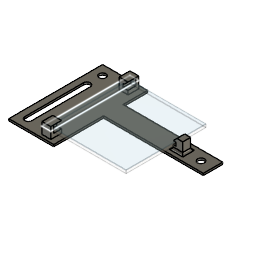
MDB-Slave-PCB-Holder (Autodesk Fusion 360 design; units mm, degrees)
Autodesk Fusion 360 part; units mm, degrees
sketch "Skizze1" plane through (0, 0, 0) normal (0, 0, 1) x (1, 0, 0) in component "Component"
  line L0 (19.5, -20.5) -> (-19.5, -20.5)
  line L1 (-19.5, -20.5) -> (-19.5, 20.5)
  line L2 (-19.5, 20.5) -> (19.5, 20.5)
  line L3 (19.5, 20.5) -> (19.5, -20.5)
  line L4 (19.5, -20.5) -> (-19.5, 20.5) construction
  line L5 (-19.5, -20.5) -> (19.5, 20.5) construction
  dimension "d19" = 39
  dimension "d20" = 41
  constraint horizontal L0
  constraint perpendicular L0 L1
  constraint parallel L0 L2
  constraint parallel L1 L3
  constraint coincident L4 origin
  constraint coincident L5 origin
  measures "d19" distance of L1.end L2.end
  measures "d20" distance of L0.end L1.end
extrude "Extrusion1" add sketch "Skizze1" along normal blind 1.7 makes body 1 in component "Component"
sketch "Skizze1 (2)" plane through (0, 0, 1.7) normal (0, 0, 1) x (-1, 0, 0) in component "Component'"
  line L0 (-19.5, -20.5) -> (19.5, -20.5)
  line L1 (19.5, -20.5) -> (19.5, 20.5)
  line L2 (19.5, 20.5) -> (-19.5, 20.5)
  line L3 (-19.5, 20.5) -> (-19.5, -20.5)
  line L4 (17, -22.5) -> (21.5, -22.5)
  line L5 (21.5, -22.5) -> (21.5, 22.5)
  line L6 (21.5, 22.5) -> (17, 22.5)
  line L7 (17, 22.5) -> (17, -22.5)
  dimension "d23" = 2
  dimension "d24" = 2
  dimension "d25" = 2.5
  dimension "d26" = 2
  constraint horizontal L4
  constraint vertical L5
  constraint horizontal L6
  constraint vertical L7
  measures "d23" distance of L2 L6
  measures "d24" distance of L0 L4
  measures "d25" distance of L1 L7
  measures "d26" distance of L1 L5
extrude "Extrusion1'" add sketch "Skizze1 (2)" against normal up to surface (1.7 mm away) separate body contours L0 L1 L2 L4 L5 L6 L7 makes body 2 in component "Component'"
extrude "Extrusion2" add sketch "Skizze1 (2)" along normal blind 1 separate body contours L0 L1 L2 L7 | L0 L1 L2 L4 L5 L6 L7 makes body 3 in component "Component'"
sketch "Skizze2" plane through (0, 0, 0) normal (0, 0, -1) x (1, 0, 0) in component "Component'"
  line L0 (-21.5, -22.5) -> (-17, -22.5)
  line L1 (-17, -22.5) -> (-17, -20.5)
  line L2 (-17, -20.5) -> (-19.5, -20.5)
  line L3 (-19.5, -20.5) -> (-19.5, 20.5)
  line L4 (-19.5, 20.5) -> (-17, 20.5)
  line L5 (-17, 20.5) -> (-17, 22.5)
  line L6 (-17, 22.5) -> (-21.5, 22.5)
  line L7 (-21.5, 22.5) -> (-21.5, -22.5)
  line L8 (-17, -20.5) -> (-17, 20.5)
  constraint coincident L1.end L2.start
  constraint coincident L4.end L5.start
extrude "Extrusion3" add sketch "Skizze2" along normal blind 2 bodies 2 in component "Component'"
sketch "Skizze3" plane through (0, 0, -2) normal (0, 0, -1) x (1, 0, 0) in component "Component'"
  line L0 (-17, -22.5) -> (-17, 22.5)
  line L1 (-17, 22.5) -> (-21.5, 22.5)
  line L2 (-21.5, 22.5) -> (-21.5, -22.5)
  line L3 (-21.5, -22.5) -> (-17, -22.5)
  line L4 (27, -24) -> (-27, -24)
  line L5 (-27, -24) -> (-27, 24)
  line L6 (-27, 24) -> (27, 24)
  line L7 (27, 24) -> (27, -24)
  line L8 (27, -24) -> (-27, 24) construction
  line L9 (-27, -24) -> (27, 24) construction
  constraint horizontal L4
  constraint perpendicular L4 L5
  constraint parallel L4 L6
  constraint parallel L5 L7
  constraint coincident L8 origin
  constraint coincident L9 origin
extrude "Extrusion4" add sketch "Skizze3" along normal blind 1 contours L0 L1 L2 L3 | L4 L5 L6 L7 bodies 2 in component "Component'"
sketch "Skizze4" plane through (0, 0, -2) normal (0, 0, 1) x (-1, 0, 0) in component "Component'"
  line L0 (27, 24) -> (-27, 24)
  line L1 (-27, 24) -> (-27, -24)
  line L2 (-27, -24) -> (27, -24)
  line L3 (27, -24) -> (27, 24)
  line L4 (21.5, -22.5) -> (17, -22.5)
  line L5 (17, -22.5) -> (17, 22.5)
  line L6 (17, 22.5) -> (21.5, 22.5)
  line L7 (21.5, 22.5) -> (21.5, -22.5)
  line L8 (-23.5, -8.5) -> (-18.5, -8.5)
  line L9 (-18.5, -8.5) -> (-18.5, -4.5)
  line L10 (-18.5, -4.5) -> (-23.5, -4.5)
  line L11 (-23.5, -4.5) -> (-23.5, -8.5)
  line L12 (-19.5, -20.5) -> (19.5, -20.5)
  line L13 (-19.5, 20.5) -> (-19.5, -20.5)
  dimension "d35" = 12
  dimension "d36" = 4
  dimension "d37" = 4
  dimension "d38" = 1
  constraint horizontal L8
  constraint vertical L9
  constraint horizontal L10
  constraint vertical L11
  measures "d35" distance of L8 L12
  measures "d36" distance of L8.start L10.end
  measures "d37" distance of L11 L13
  measures "d38" distance of L9 L13
extrude "Extrusion5" add sketch "Skizze4" along normal up to surface (5.7 mm away) contours L8 L10 L11 L13 | L8 L9 L10 L13 bodies 2 in component "Component'"
chamfer "Fase1" distance 2 angle 45 1 edges at (18.5, 6.5, 3.7) on bodies 2 in component "Component'"
extrude "Extrusion6" cut 1 faces at (19.5, -6.8333, 1.1333) along direction (-1, 0, 0) blind 2 on bodies 1 bodies 2 in component "Component'"
extrude "Extrusion7" cut 1 faces at (19.5, 7.1667, 0.5667) along direction (1, 0, 0) blind 0.5 on bodies 2 bodies 2 in component "Component'"
fillet "Abrundung1" radius 1 4 edges at (21, 4.5, -2) (23.5, 6.5, -2) (18.5, 6.5, -2) (21, 8.5, -2) on bodies 2 in component "Component'"
extrude "Extrusion8" add 1 faces at (-20, 6.8333, 2.7) along direction (0, 0, 1) blind 1 on bodies 3 bodies 3 in component "Component'"
chamfer "Fase2" distance 2 angle 45 1 edges at (-17, 0, 1.7) on bodies 3 in component "Component'"
extrude "Extrusion9" add sketch "Skizze1 (2)" along normal up to surface (2 mm away) contours L0 L1 L2 L4 L5 L6 L7 bodies 2 3 in component "Component'"
sketch "Skizze5" plane through (0, 0, -2) normal (0, 0, 1) x (-1, 0, 0) in component "Component'"
  line L0 (21.5, -22.5) -> (17, -22.5)
  line L1 (17, -22.5) -> (17, 22.5)
  line L2 (17, 22.5) -> (21.5, 22.5)
  line L3 (21.5, 22.5) -> (21.5, -22.5)
  line L4 (27, 24) -> (-27, 24)
  line L5 (-27, 24) -> (-27, -24)
  line L6 (-27, -24) -> (27, -24)
  line L7 (27, -24) -> (27, 24)
  line L8 (-24.5, -3.5) -> (-17.5, -3.5)
  line L9 (-17.5, -3.5) -> (-17.5, -9.5)
  line L10 (-17.5, -9.5) -> (-24.5, -9.5)
  line L11 (-24.5, -9.5) -> (-24.5, -3.5)
  line L12 (-27, 24) -> (14, 24)
  line L13 (14, 24) -> (14, -1.5)
  line L14 (14, -1.5) -> (-27, -1.5)
  line L15 (-27, -1.5) -> (-27, 24)
  line L16 (-27, -24) -> (14, -24)
  line L17 (14, -24) -> (14, -11.5)
  line L18 (14, -11.5) -> (-27, -11.5)
  line L19 (-27, -11.5) -> (-27, -24)
  line L20 (17, 20.5) -> (17, -20.5)
  dimension "d65" = 2
  dimension "d66" = 2
  dimension "d67" = 3
  dimension "d68" = 3
  constraint horizontal L12
  constraint vertical L13
  constraint horizontal L14
  constraint vertical L15
  constraint coincident L4.end L5.start
  constraint horizontal L16
  constraint vertical L17
  constraint horizontal L18
  constraint vertical L19
  constraint coincident L5.end L6.start
  measures "d65" distance of L10 L18
  measures "d66" distance of L8 L14
  measures "d67" distance of L13 L20
  measures "d68" distance of L17 L20
extrude "Extrusion10" cut sketch "Skizze5" against normal up to surface (1 mm away) contours L4 L5 L12 L13 L14 L15 | L5 L6 L16 L17 L18 L19 bodies 2 in component "Component'"
extrude "Extrusion11" cut 1 faces at (19.5, 7.1667, 1.7) along direction (0, 0, 1) blind 0.2 on bodies 2 bodies 2 in component "Component'"
fillet "Abrundung2" radius 0.5 1 edges at (20, 6.5, 1.9) on bodies 2 in component "Component'"
sketch "Skizze6" plane through (0, 0, 3.7) normal (0, 0, 1) x (-1, 0, 0) in component "Component'"
  line L0 (17, -20.5) -> (17, -22.5)
  line L1 (17, -22.5) -> (21.5, -22.5)
  line L2 (21.5, -22.5) -> (21.5, 22.5)
  line L3 (21.5, 22.5) -> (17, 22.5)
  line L4 (17, 22.5) -> (17, 20.5)
  line L5 (17, 20.5) -> (17, -20.5)
  line L6 (12, 17) -> (26, 17)
  line L7 (26, 17) -> (26, -17)
  line L8 (26, -17) -> (12, -17)
  line L9 (12, -17) -> (12, 17)
  line L10 (12, 17) -> (26, -17) construction
  line L11 (26, 17) -> (12, -17) construction
  point P0 (19, 0)
  constraint horizontal L6
  constraint perpendicular L6 L7
  constraint parallel L6 L8
  constraint parallel L7 L9
  constraint coincident L10 P0
  constraint coincident L11 P0
extrude "Extrusion12" cut sketch "Skizze6" against normal up to surface (5.7 mm away) contours L2 L5 L6 L8 bodies 2 in component "Component'"
extrude "Extrusion13" cut 1 faces at (-17.6665, 20.5, 1.7999) along direction (0, 1, 0) blind 0.5 on bodies 2 bodies 2 in component "Component'"
extrude "Extrusion14" cut 1 faces at (-17.6665, -20.5, 1.7999) along direction (0, -1, 0) blind 0.5 on bodies 2 bodies 2 in component "Component'"
extrude "Extrusion15" add 1 faces at (27, 4.8333, -2.3333) along direction (1, 0, 0) blind 10 on bodies 2 bodies 2 in component "Component'"
extrude "Extrusion16" add 1 faces at (-27, 8, -2.3333) along direction (-1, 0, 0) blind 10 on bodies 2 bodies 2 in component "Component'"
sketch "Skizze7" plane through (0, 0, -2) normal (0, 0, 1) x (-1, 0, 0) in component "Component'"
  line L0 (21.5, -17) -> (21.5, -22.5)
  line L1 (21.5, -22.5) -> (17, -22.5)
  line L2 (17, -22.5) -> (17, -17)
  line L3 (17, -17) -> (21.5, -17)
  line L4 (14, -11.5) -> (14, -24)
  line L5 (14, -24) -> (37, -24)
  line L6 (37, -24) -> (37, 24)
  line L7 (37, 24) -> (14, 24)
  line L8 (14, 24) -> (14, -1.5)
  line L9 (14, -1.5) -> (-37, -1.5)
  line L10 (-37, -1.5) -> (-37, -11.5)
  line L11 (-37, -11.5) -> (14, -11.5)
  line L12 (21.5, 17) -> (17, 17)
  line L13 (17, 17) -> (17, 22.5)
  line L14 (17, 22.5) -> (21.5, 22.5)
  line L15 (21.5, 22.5) -> (21.5, 17)
  line L16 (-17.5, -9.5) -> (-24.5, -9.5)
  line L17 (-24.5, -9.5) -> (-24.5, -3.5)
  line L18 (-24.5, -3.5) -> (-17.5, -3.5)
  line L19 (-17.5, -3.5) -> (-17.5, -9.5)
  circle A0 centre (-30.8617, -6.5) radius 1.75
  line L20 (-24.7234, -1.5) -> (-37, -11.5) construction
  line L21 (-24.7234, -11.5) -> (-37, -1.5) construction
  circle A1 centre (32, -19) radius 1.75
  line L22 (33.75, -11) -> (33.75, 19)
  arc A2 (33.75, 19) -> (30.25, 19) centre (32, 19) ccw
  line L23 (30.25, 19) -> (30.25, -11)
  arc A3 (30.25, -11) -> (33.75, -11) centre (32, -11) ccw
  line L24 (32, -11) -> (32, 19) construction
  dimension "d74" = 3.5
  dimension "d75" = 3.5
  dimension "d76" = 5
  dimension "d77" = 3.5
  dimension "d78" = 8
  dimension "d79" = 5
  dimension "d80" = 5
  dimension "d81" = 5
  constraint coincident L9 L20.start
  constraint coincident L10.end L11.start
  constraint coincident L11 L21.start
  constraint coincident L9.end L10.start
  constraint midpoint A0.centre L20
  constraint tangent L22 A2
  constraint tangent A2 L23
  constraint parallel L22 L23
  constraint tangent L23 A3
  constraint tangent L22 A3
  constraint vertical L24
  measures "d74" diameter of A0
  measures "d75" diameter of A1
  measures "d76" distance of L6 A1.centre
  measures "d77" diameter of A2
  measures "d78" distance of A1.centre A3.centre
  measures "d79" distance of L5 A1.centre
  measures "d80" distance of L7 A2.centre
  measures "d81" distance of L6 A2.centre
extrude "Extrusion17" cut sketch "Skizze7" against normal up to surface (1 mm away) contours A0 | A1 | L22 A2 L23 A3 bodies 2 in component "Component'"
component "Component" placed x (1, 0, 0) y (0, 1, 0) z (0, 0, 1) at (0, 0, 0)
component "Component'" placed x (1, 0, 0) y (0, 1, 0) z (0, 0, 1) at (0, 0, 0)
